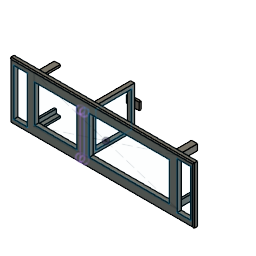
Titan_Dash_Panel_1 test 1 - (Autodesk Fusion 360 design; units mm, degrees)
part number: 2026-08-09-09-25-20-493
Autodesk Fusion 360 part; units mm, degrees
sketch "Sketch1" plane through (0, 0, 0) normal (0, 0, 1) x (1, 0, 0)
  line L0 (115.57, 35.56) -> (-115.57, 35.56)
  line L1 (-115.57, 35.56) -> (-115.57, -35.56)
  line L2 (-115.57, -35.56) -> (115.57, -35.56)
  line L3 (115.57, -35.56) -> (115.57, 35.56)
  line L4 (115.57, 35.56) -> (-115.57, -35.56) construction
  line L5 (-115.57, 35.56) -> (115.57, -35.56) construction
  dimension "d8" = 231.14
  dimension "d9" = 71.12
  constraint horizontal L0
  constraint perpendicular L0 L1
  constraint parallel L0 L2
  constraint parallel L1 L3
  constraint coincident L4 origin
  constraint coincident L5 origin
  measures "d8" distance of L1.end L2.end
  measures "d9" distance of L0.end L1.end
extrude "Extrude1" add sketch "Sketch1" along normal blind 5.08
fillet "Fillet1" radius 1.27 4 edges at (-115.57, 0, 5.08) (0, 35.56, 5.08) (115.57, 0, 5.08) (0, -35.56, 5.08)
sketch "Sketch2" plane through (0, 0, 0) normal (0, 0, -1) x (-1, 0, 0)
  line L0 (-115.57, 35.56) -> (-115.57, -35.56)
  line L1 (-115.57, -35.56) -> (115.57, -35.56)
  line L2 (115.57, -35.56) -> (115.57, 35.56)
  line L3 (115.57, 35.56) -> (-115.57, 35.56)
  line L4 (90.17, -29.21) -> (-90.17, -29.21)
  line L5 (-90.17, -29.21) -> (-90.17, 29.21)
  line L6 (-90.17, 29.21) -> (90.17, 29.21)
  line L7 (90.17, 29.21) -> (90.17, -29.21)
  line L8 (90.17, -29.21) -> (-90.17, 29.21) construction
  line L9 (-90.17, -29.21) -> (90.17, 29.21) construction
  line L10 (21.9978, -29.21) -> (27.0778, -29.21)
  line L11 (27.0778, -29.21) -> (27.0778, 22.86)
  line L12 (27.0778, 22.86) -> (21.9978, 22.86)
  line L13 (21.9978, 22.86) -> (21.9978, -29.21)
  dimension "d14" = 180.34
  dimension "d15" = 58.42
  dimension "d39" = 5.08
  constraint horizontal L4
  constraint perpendicular L4 L5
  constraint parallel L4 L6
  constraint parallel L5 L7
  constraint coincident L8 origin
  constraint coincident L9 origin
  constraint horizontal L10
  constraint vertical L11
  constraint horizontal L12
  constraint vertical L13
  constraint coincident L4 L10.start
  measures "d14" distance of L5.end L6.end
  measures "d15" distance of L4.end L5.end
  measures "d39" distance of L10.start L10.end
sketch "Sketch3" plane through (0, 0, 0) normal (0, 0, -1) x (-1, 0, 0)
sketch "Sketch4" plane through (0, 0, 0) normal (0, 0, -1) x (-1, 0, 0)
  line L0 (-90.17, 29.21) -> (90.17, 29.21)
  line L1 (-90.17, -29.21) -> (-90.17, 29.21)
  line L2 (90.17, -29.21) -> (-90.17, -29.21)
  line L3 (90.17, 29.21) -> (90.17, -29.21)
  line L4 (-90.17, 29.21) -> (-82.55, 29.21)
  line L5 (-82.55, 29.21) -> (-82.55, 26.67)
  line L6 (-82.55, 26.67) -> (-90.17, 26.67)
  line L7 (-90.17, 26.67) -> (-90.17, 29.21)
  line L8 (-90.17, 29.21) -> (-87.63, 29.21)
  line L9 (-87.63, 29.21) -> (-87.63, 21.59)
  line L10 (-87.63, 21.59) -> (-90.17, 21.59)
  line L11 (-90.17, 21.59) -> (-90.17, 29.21)
  line L12 (-90.17, -29.21) -> (-87.63, -29.21)
  line L13 (-87.63, -29.21) -> (-87.63, -21.59)
  line L14 (-87.63, -21.59) -> (-90.17, -21.59)
  line L15 (-90.17, -21.59) -> (-90.17, -29.21)
  line L16 (-90.17, -29.21) -> (-87.63, -29.21)
  line L17 (-87.63, -29.21) -> (-87.63, -21.59)
  line L18 (-87.63, -21.59) -> (-90.17, -21.59)
  line L19 (-90.17, -21.59) -> (-90.17, -29.21)
  line L20 (-90.17, -29.21) -> (-82.55, -29.21)
  line L21 (-82.55, -29.21) -> (-82.55, -26.67)
  line L22 (-82.55, -26.67) -> (-90.17, -26.67)
  line L23 (-90.17, -26.67) -> (-90.17, -29.21)
  line L24 (90.17, 29.21) -> (82.55, 29.21)
  line L25 (82.55, 29.21) -> (82.55, 26.67)
  line L26 (82.55, 26.67) -> (90.17, 26.67)
  line L27 (90.17, 26.67) -> (90.17, 29.21)
  line L28 (90.17, 29.21) -> (87.63, 29.21)
  line L29 (87.63, 29.21) -> (87.63, 21.59)
  line L30 (87.63, 21.59) -> (90.17, 21.59)
  line L31 (90.17, 21.59) -> (90.17, 29.21)
  line L32 (90.17, -29.21) -> (87.63, -29.21)
  line L33 (87.63, -29.21) -> (87.63, -21.59)
  line L34 (87.63, -21.59) -> (90.17, -21.59)
  line L35 (90.17, -21.59) -> (90.17, -29.21)
  line L36 (90.17, -29.21) -> (82.55, -29.21)
  line L37 (82.55, -29.21) -> (82.55, -26.67)
  line L38 (82.55, -26.67) -> (90.17, -26.67)
  line L39 (90.17, -26.67) -> (90.17, -29.21)
  dimension "d17" = 7.62
  dimension "d18" = 2.54
  dimension "d19" = 2.54
  dimension "d20" = 7.62
  dimension "d21" = 2.54
  dimension "d22" = 7.62
  dimension "d23" = 2.54
  dimension "d24" = 7.62
  dimension "d25" = 7.62
  dimension "d26" = 2.54
  dimension "d27" = 7.62
  dimension "d28" = 2.54
  dimension "d29" = 2.54
  dimension "d30" = 7.62
  dimension "d31" = 2.54
  dimension "d32" = 7.62
  dimension "d33" = 7.62
  dimension "d34" = 2.54
  constraint horizontal L4
  constraint vertical L5
  constraint horizontal L6
  constraint vertical L7
  constraint coincident L0.start L1.end
  constraint horizontal L8
  constraint vertical L9
  constraint horizontal L10
  constraint vertical L11
  constraint horizontal L12
  constraint vertical L13
  constraint horizontal L14
  constraint vertical L15
  constraint coincident L1.start L2.end
  constraint horizontal L16
  constraint vertical L17
  constraint horizontal L18
  constraint vertical L19
  constraint horizontal L20
  constraint vertical L21
  constraint horizontal L22
  constraint vertical L23
  constraint horizontal L24
  constraint vertical L25
  constraint horizontal L26
  constraint vertical L27
  constraint coincident L0.end L3.start
  constraint horizontal L28
  constraint vertical L29
  constraint horizontal L30
  constraint vertical L31
  constraint horizontal L32
  constraint vertical L33
  constraint horizontal L34
  constraint vertical L35
  constraint coincident L2.start L3.end
  constraint horizontal L36
  constraint vertical L37
  constraint horizontal L38
  constraint vertical L39
  measures "d17" distance of L0.start L4.end
  measures "d18" distance of L0.start L6.end
  measures "d19" distance of L0.start L8.end
  measures "d20" distance of L0.start L10.end
  measures "d21" distance of L1.start L12.end
  measures "d22" distance of L1.start L14.end
  measures "d23" distance of L1.start L12.end
  measures "d24" distance of L1.start L14.end
  measures "d25" distance of L1.start L20.end
  measures "d26" distance of L1.start L22.end
  measures "d27" distance of L0.end L24.end
  measures "d28" distance of L0.end L26.end
  measures "d29" distance of L0.end L28.end
  measures "d30" distance of L0.end L30.end
  measures "d31" distance of L2.start L32.end
  measures "d32" distance of L2.start L34.end
  measures "d33" distance of L2.start L36.end
  measures "d34" distance of L2.start L38.end
extrude "Extrude2" add sketch "Sketch4" along normal blind 25.4 contours L0 L1 L4 L6 L7 L8 L9 L11 | L0 L4 L5 L6 L9 | L1 L6 L9 L10 L11 | L0 L24 L25 L26 L29 | L1 L13 L14 L15 L17 L18 L19 L22 | L0 L3 L24 L26 L27 L28 L29 L31 | L1 L2 L12 L13 L15 L16 L17 L19 L20 L22 L23 | L3 L26 L29 L30 L31 | L2 L13 L17 L20 L21 L22 | L3 L33 L34 L35 L38 | L2 L33 L36 L37 L38 | L2 L3 L32 L33 L35 L36 L38 L39
extrude "Extrude4" add sketch "Sketch2" along normal blind 58.42 contours L4 L10 L11 L12 L13
sketch "Sketch5" plane through (0, 0, -58.42) normal (0, 0, -1) x (-1, 0, 0)
  line L0 (21.9978, 22.86) -> (21.9978, -29.21)
  line L1 (21.9978, -29.21) -> (27.0778, -29.21)
  line L2 (27.0778, -29.21) -> (27.0778, 22.86)
  line L3 (27.0778, 22.86) -> (21.9978, 22.86)
  line L4 (32.5415, -4.6498) -> (16.3444, -4.6498)
  line L5 (16.3444, -4.6498) -> (16.3444, 4.6993)
  line L6 (16.3444, 4.6993) -> (32.5415, 4.6993)
  line L7 (32.5415, 4.6993) -> (32.5415, -4.6498)
  line L8 (32.5415, -4.6498) -> (16.3444, 4.6993) construction
  line L9 (16.3444, -4.6498) -> (32.5415, 4.6993) construction
  point P0 (24.443, 0.0247)
  constraint horizontal L4
  constraint perpendicular L4 L5
  constraint parallel L4 L6
  constraint parallel L5 L7
  constraint coincident L8 P0
  constraint coincident L9 P0
extrude "Extrude5" add sketch "Sketch5" along normal blind 2.54 contours L0 L2 L4 L6 | L0 L4 L5 L6 | L2 L4 L6 L7
sketch "Sketch6" plane through (0, 0, 5.08) normal (0, 0, 1) x (1, 0, 0)
  line L0 (114.3, -34.29) -> (114.3, 34.29)
  line L1 (114.3, 34.29) -> (-114.3, 34.29)
  line L2 (-114.3, 34.29) -> (-114.3, -34.29)
  line L3 (-114.3, -34.29) -> (114.3, -34.29)
  line L4 (-27.0778, -29.21) -> (-27.0778, 22.86)
  line L5 (-21.9978, 22.86) -> (-21.9978, -29.21)
  line L6 (-84.4681, 24.2382) -> (-31.4836, 24.2382)
  line L7 (-31.4836, 24.2382) -> (-31.4836, -22.6712)
  line L8 (-31.4836, -22.6712) -> (-84.4681, -22.6712)
  line L9 (-84.4681, -22.6712) -> (-84.4681, 24.2382)
  line L10 (-15.8698, 24.4915) -> (84.98, 24.4915)
  line L11 (84.98, 24.4915) -> (84.98, -23.4013)
  line L12 (84.98, -23.4013) -> (-15.8698, -23.4013)
  line L13 (-15.8698, -23.4013) -> (-15.8698, 24.4915)
  line L14 (111.9771, 30.423) -> (95.1039, 30.423)
  line L15 (95.1039, 30.423) -> (95.1039, -28.1221)
  line L16 (95.1039, -28.1221) -> (111.9771, -28.1221)
  line L17 (111.9771, -28.1221) -> (111.9771, 30.423)
  line L18 (-93.8256, 29.4004) -> (-110.6989, 29.4004)
  line L19 (-110.6989, 29.4004) -> (-110.6989, -29.4004)
  line L20 (-110.6989, -29.4004) -> (-93.8256, -29.4004)
  line L21 (-93.8256, -29.4004) -> (-93.8256, 29.4004)
  constraint horizontal L6
  constraint vertical L7
  constraint horizontal L8
  constraint vertical L9
  constraint horizontal L10
  constraint vertical L11
  constraint horizontal L12
  constraint vertical L13
  constraint horizontal L14
  constraint vertical L15
  constraint horizontal L16
  constraint vertical L17
  constraint horizontal L18
  constraint vertical L19
  constraint horizontal L20
  constraint vertical L21
extrude "Extrude6" cut sketch "Sketch6" against normal blind 12.7 contours L6 L7 L8 L9 | L10 L11 L12 L13 | L14 L15 L16 L17 | L18 L19 L20 L21
sketch "Sketch7" plane through (-21.9978, 0, 0) normal (1, 0, 0) x (0, 0, -1)
  line L0 (0, 22.86) -> (0, -29.21)
  line L1 (0, -29.21) -> (58.42, -29.21)
  line L2 (58.42, -29.21) -> (58.42, -4.6498)
  line L3 (58.42, -4.6498) -> (58.42, 4.6993)
  line L4 (58.42, 4.6993) -> (58.42, 22.86)
  line L5 (58.42, 22.86) -> (0, 22.86)
  line L6 (9.4593, 18.1515) -> (54.199, 18.1515)
  line L7 (54.199, 18.1515) -> (54.199, -25.8212)
  line L8 (54.199, -25.8212) -> (9.4593, -25.8212)
  line L9 (9.4593, -25.8212) -> (9.4593, 18.1515)
  constraint horizontal L6
  constraint vertical L7
  constraint horizontal L8
  constraint vertical L9
extrude "Extrude7" cut sketch "Sketch7" against normal blind 7.62 contours L6 L7 L8 L9
sketch "Sketch8" plane through (0, 0, 5.08) normal (0, 0, 1) x (1, 0, 0)
extrude "Extrude3" [rolled back] along distance 58.42 taper angle 0
equation "panelWidth = innerWidth + 2 * widthMargin"
equation "panelHeight = innerHeight + heightMargin"
equation "panelThickness = 0.2 in"
equation "panelFrontFillet = 0.05 in"
equation "bossThickness = 0.1 in"
equation "innerWidth = 7.1 in"
equation "innerHeight = 2.3 in"
equation "d8 = panelWidth"
equation "d9 = panelHeight"
equation "d10 = panelThickness"
equation "d13 = panelFrontFillet"
equation "d14 = innerWidth"
equation "d15 = innerHeight"
equation "bossWidth = 0.3 in"
equation "d17 = bossWidth"
equation "d18 = bossThickness"
equation "d19 = bossThickness"
equation "d20 = bossWidth"
equation "d21 = bossThickness"
equation "d22 = bossWidth"
equation "d23 = bossThickness"
equation "d24 = bossWidth"
equation "d25 = bossWidth"
equation "d26 = bossThickness"
equation "d27 = bossWidth"
equation "d28 = bossThickness"
equation "d29 = bossThickness"
equation "d30 = bossWidth"
equation "d31 = bossThickness"
equation "d32 = bossWidth"
equation "d33 = bossWidth"
equation "d34 = bossThickness"
equation "widthMargin = 1 in"
equation "heightMargin = 0.5 in"
